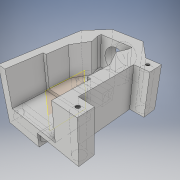
# Autodesk Inventor part: AC_wire_holder
Saved by Autodesk Inventor 2019 (Build 230136000, 136)
## iProperties
Created: 2019-08-30
Part Number: AC_wire_holder
Material: Generic
Document SubType Name: Modeling
Designer: fablab
Density: 1 g/cm^3
Appearance: Default
Author: fablab
Autodesk Inventor part; units mm, degrees
ref_plane "YZ Plane" through (0, 0, 0) normal (1, 0, 0) x (0, 1, 0)
ref_plane "XZ Plane" through (0, 0, 0) normal (0, 1, 0) x (-1, 0, 0)
ref_plane "XY Plane" through (0, 0, 0) normal (0, 0, 1) x (1, 0, 0)
sketch "Sketch1" plane through (0, 0, 0) normal (0, 1, 0) x (-1, 0, 0)
  line L0 (0, 0) -> (-25.32, 0)
  line L1 (-25.32, 0) -> (-25.32, -13)
  line L2 (-25.32, -13) -> (0, -13)
  line L3 (0, -13) -> (0, 0)
  dimension "d0" = 25.32
  dimension "d1" = 13
  constraints: 8 end point, 2 parallel, 1 horizontal, 1 perpendicular
  measures "d0" distance of L2.end L1.end
  measures "d1" distance of L1.end L0.end
extrude "Extrusion1" add sketch "Sketch1" along normal blind 5
sketch "Sketch2" plane through (25.32, 0, 0) normal (1, 0, 0) x (0, 0, -1)
  line L0 (0, 0) -> (13, 0)
  line L1 (13, 0) -> (13, 21.3)
  line L2 (13, 21.3) -> (0, 21.3)
  line L3 (0, 21.3) -> (0, 0)
  dimension "d4" = 13
  dimension "d5" = 21.3
  constraints: 8 end point, 2 parallel, 1 horizontal, 1 perpendicular
  measures "d4" distance of L2.end L1.end
  measures "d5" distance of L1.end L0.end
extrude "Extrusion2" add sketch "Sketch2" along normal blind 7
sketch "Sketch3" plane through (0, 0, 0) normal (0, -1, 0) x (1, 0, 0)
  line L0 (25.32, -13) -> (0, -13) projected
  line L1 (25.32, -8.0084) -> (25.32, -13)
  line L2 (25.32, -13) -> (25.32, -23) construction
  line L3 (25.32, -23) -> (20.12, -23) construction
  line L4 (20.12, -23) -> (25.32, -13)
  line L5 (20.12, -23) -> (5.2, -23)
  line L6 (0, -23) -> (5.2, -23)
  line L7 (5.2, -23) -> (0, -13)
  line L8 (0, -13) -> (5.2, -23)
  point P0 (0, 0)
  dimension "d8" = 10
  dimension "d9" = 5.2
  dimension "d10" = 5.2
  constraints: 16 end point, 2 horizontal, 1 collinear, 1 point on line, 1 vertical
  measures "d8" distance of L0.start L2.end
  measures "d9" distance of L2.end L3.end
  measures "d10" distance of L5.end L6.start
extrude "Extrusion3" add sketch "Sketch3" against normal blind 5
sketch "Sketch4" plane through (0, 0, 0) normal (0, -1, 0) x (1, 0, 0)
  line L0 (20.12, -23) -> (25.32, -13) projected
  line L1 (20.12, -23) -> (27.32, -23)
  line L2 (25.32, -13) -> (32.32, -13) projected
  line L3 (32.32, -13) -> (27.32, -23)
  point P0 (0, 0)
  dimension "d13" = 7.2
  constraints: 4 end point, 1 horizontal
  measures "d13" distance of L0.start L1.end
extrude "Extrusion4" add sketch "Sketch4" against normal blind 21.3
sketch "Sketch5" plane through (0, 0, 0) normal (0, -1, 0) x (1, 0, 0)
  line L0 (20.12, -23) -> (5.2, -23) projected
  line L1 (20.12, -23) -> (20.12, -28.9) construction
  line L2 (20.12, -28.9) -> (22.12, -28.9) construction
  line L3 (20.12, -23) -> (25.32, -13) projected
  line L4 (22.12, -28.9) -> (20.12, -23)
  line L5 (27.32, -23) -> (20.12, -23) projected
  line L6 (27.32, -23) -> (27.32, -28.9)
  line L7 (27.32, -28.9) -> (29.32, -28.9) construction
  line L8 (29.32, -28.9) -> (27.32, -23)
  line L9 (29.32, -28.9) -> (22.12, -28.9)
  line L10 (5.2, -23) -> (5.2, -28.9) construction
  line L11 (5.2, -28.9) -> (3.2, -28.9) construction
  line L12 (3.2, -28.9) -> (5.2, -23)
  line L13 (22.12, -28.9) -> (3.2, -28.9)
  point P0 (0, 0)
  dimension "d16" = 5.9
  dimension "d17" = 2
  dimension "d18" = 2
  dimension "d19" = 2
  constraints: 22 end point, 2 collinear, 2 perpendicular, 2 point on line, 2 vertical, 1 horizontal
  measures "d16" distance of L0.start L1.end
  measures "d17" distance of L1.end L2.end
  measures "d18" distance of L6.end L7.end
  measures "d19" distance of L10.end L11.end
extrude "Extrusion5" add sketch "Sketch5" against normal blind 5 contours L4 L13 L12 L0
sketch "Sketch6" plane through (0, 0, 0) normal (0, -1, 0) x (1, 0, 0)
  line L0 (20.12, -23) -> (27.32, -23) projected
  line L1 (27.32, -23) -> (27.32, -28.9) construction
  line L2 (27.32, -28.9) -> (29.32, -28.9) construction
  line L3 (29.32, -28.9) -> (27.32, -23)
  line L4 (20.12, -23) -> (22.12, -28.9) projected
  line L5 (29.32, -28.9) -> (22.12, -28.9)
  point P0 (0, 0)
  dimension "d22" = 5.9
  dimension "d23" = 2
  constraints: 8 end point, 1 perpendicular, 1 vertical
  measures "d22" distance of L0.end L1.end
  measures "d23" distance of L1.end L2.end
extrude "Extrusion6" add sketch "Sketch6" against normal blind 21.3
sketch "Sketch7" plane through (0, 0, 0) normal (0, -1, 0) x (1, 0, 0)
  line L0 (22.12, -28.9) -> (3.2, -28.9) projected
  line L1 (22.12, -28.9) -> (22.12, -31.4)
  line L2 (3.2, -28.9) -> (5.2, -23) projected
  line L3 (3.2, -28.9) -> (3.2, -31.4)
  line L4 (3.2, -31.4) -> (22.12, -31.4)
  point P0 (0, 0)
  dimension "d26" = 2.5
  dimension "d27" = 2.5
  constraints: 6 end point, 2 vertical
  measures "d26" distance of L0.start L1.end
  measures "d27" distance of L0.end L3.end
extrude "Extrusion7" add sketch "Sketch7" against normal blind 5
sketch "Sketch8" plane through (0, 0, 0) normal (0, -1, 0) x (1, 0, 0)
  line L0 (27.32, -23) -> (29.32, -28.9) projected
  line L1 (22.12, -28.9) -> (22.12, -31.4) projected
  line L2 (29.32, -28.9) -> (22.12, -28.9)
  line L3 (22.12, -28.9) -> (22.12, -31.4)
  line L4 (22.12, -31.4) -> (29.32, -31.4)
  line L5 (29.32, -31.4) -> (29.32, -28.9)
  point P0 (0, 0)
  constraints: 8 end point, 2 parallel, 1 horizontal, 1 perpendicular
extrude "Extrusion8" add sketch "Sketch8" against normal blind 21.3
sketch "Sketch9" plane through (0, 0, 0) normal (0, -1, 0) x (1, 0, 0)
  line L0 (22.12, -31.4) -> (3.2, -31.4) projected
  line L1 (3.2, -31.4) -> (22.12, -31.4)
  line L2 (22.12, -31.4) -> (22.12, -39.7)
  line L3 (22.12, -39.7) -> (3.2, -39.7)
  line L4 (3.2, -39.7) -> (3.2, -31.4)
  point P0 (0, 0)
  dimension "d32" = 18.92
  dimension "d33" = 8.3
  constraints: 8 end point, 2 parallel, 1 horizontal, 1 perpendicular
  measures "d32" distance of L2.end L3.end
  measures "d33" distance of L3.end L0.end
extrude "Extrusion9" add sketch "Sketch9" against normal blind 21.3
sketch "Sketch10" plane through (0, 0, 0) normal (0, -1, 0) x (1, 0, 0)
  line L0 (22.12, -31.4) -> (29.32, -31.4) projected
  line L1 (22.12, -31.4) -> (22.12, -39.7) projected
  line L2 (29.32, -31.4) -> (22.12, -39.7)
  point P0 (0, 0)
  constraints: 2 end point
extrude "Extrusion10" add sketch "Sketch10" against normal blind 21.3
sketch "Sketch11" plane through (3.2, 0, -39.7) normal (0, 0, -1) x (-1, 0, 0)
  line L0 (0, 5) -> (-2, 5) projected
  line L1 (0, 5) -> (-18.878, 5) construction
  line L2 (0, 21.3) -> (-18.92, 21.3) projected
  line L3 (-9.46, 21.3) -> (-9.439, 5) construction
  line L4 (-9.4495, 13.15) -> (0, 13.1622) construction
  line L5 (0, 0) -> (0, 21.3) projected
  circle A0 centre (-9.4495, 13.15) radius 6.625
  point P0 (3.2, 0)
  dimension "d38" = 13.25
  constraints: 6 end point, 3 midpoint, 1 centre point, 1 coincident, 1 collinear, 1 perpendicular, 1 point on line
  measures "d38" diameter of A0
extrude "Extrusion11" cut sketch "Sketch11" against normal blind 21.3
sketch "Sketch12" plane through (25.32, 21.3, 0) normal (0, 1, 0) x (1, 0, 0)
  line L0 (7, 13) -> (2, 23) projected
  line L1 (4, 31.4) -> (4, 28.9) projected
  line L2 (7, 13) -> (4, 31.4)
  line L3 (2, 23) -> (4, 28.9) projected
  line L4 (2, 23) -> (4, 28.9)
  line L5 (4, 28.9) -> (4, 31.4)
  line L6 (7, 13) -> (2, 23)
  point P0 (-25.32, 0)
  constraints: 8 end point, 1 collinear, 1 vertical
extrude "Extrusion12" add sketch "Sketch12" against normal blind 21.3
sketch "Sketch13" plane through (25.32, 21.3, 0) normal (0, 1, 0) x (1, 0, 0)
  line L0 (4, 31.4) -> (7, 13) projected
  line L1 (7, 13) -> (7, 31.4) construction
  line L2 (4, 31.4) -> (7, 27.9417)
  line L3 (4, 31.4) -> (-3.2, 39.7) projected
  line L4 (7, 27.9417) -> (7, 13)
  line L5 (7, 13) -> (4, 31.4)
  point P0 (-25.32, 0)
  constraints: 8 end point, 3 collinear, 1 point on line, 1 vertical
extrude "Extrusion13" add sketch "Sketch13" against normal blind 21.3
ref_plane "Work Plane1" through (12.66, 5, 0) normal (1, 0, 0) x (0, 1, 0)
mirror "Mirror1" about plane through (12.66, 5, 0) normal (1, 0, 0)
sketch "Sketch16" plane through (25.32, 5, 0) normal (0, 0, 1) x (1, 0, 0)
  line L0 (-20.12, 0) -> (-25.32, 0) projected
  line L1 (-25.32, 0) -> (-25.32, -2) construction
  line L2 (-25.32, -2) -> (-27.32, -2)
  line L3 (-27.32, -2) -> (-27.32, 16.3)
  line L4 (-25.32, 16.3) -> (-32.32, 16.3) projected
  line L5 (0, 0) -> (2, 0) construction
  line L6 (2, 0) -> (2, -2)
  line L7 (2, -2) -> (-25.32, -2)
  line L8 (2, 0) -> (2, 16.3)
  line L9 (-27.32, 16.3) -> (-32.32, 16.3)
  line L10 (-32.32, 16.3) -> (-32.32, -5) projected
  line L11 (-32.32, 16.3) -> (-32.32, -5)
  line L12 (-32.32, -5) -> (7, -5)
  line L13 (7, 16.3) -> (7, -5) projected
  line L14 (7, -5) -> (7, 16.3)
  line L15 (7, 16.3) -> (2, 16.3)
  line L16 (0, 16.3) -> (7, 16.3) projected
  point P0 (-25.32, -5)
  dimension "d45" = 2
  dimension "d46" = 2
  dimension "d47" = 2
  dimension "d48" = 2
  constraints: 24 end point, 4 perpendicular, 3 collinear, 2 horizontal, 2 point on line, 1 vertical
  measures "d45" distance of L0.end L1.end
  measures "d46" distance of L1.end L2.end
  measures "d47" distance of L5.start L5.end
  measures "d48" distance of L5.end L6.end
extrude "Extrusion14" add sketch "Sketch16" along normal blind 19.2
sketch "Sketch22" plane through (-7, 0, -27.9417) normal (-1, 0, 0) x (0, 0, 1)
  line L0 (-11.7583, 0) -> (0, 0) projected
  line L1 (0, 0) -> (8, 0)
  line L2 (8, 0) -> (8, -8)
  line L3 (8, -8) -> (0, -8)
  line L4 (0, -8) -> (0, 0)
  line L5 (47.1417, 0) -> (0, 0) projected
  line L6 (47.1417, 0) -> (39.1417, 0)
  line L7 (39.1417, 0) -> (39.1417, -8)
  line L8 (39.1417, -8) -> (47.1417, -8)
  line L9 (47.1417, -8) -> (47.1417, 0)
  line L10 (0, -4) -> (47.1417, -4) construction
  line L11 (4, -8) -> (4, -4) construction
  line L12 (43.1417, -8) -> (43.1417, -4) construction
  circle A0 centre (4, -4) radius 1
  circle A1 centre (43.1417, -4) radius 1
  point P0 (27.9417, 0)
  dimension "d81" = 8
  dimension "d82" = 8
  dimension "d83" = 8
  dimension "d84" = 8
  dimension "d85" = 2
  dimension "d86" = 2
  constraints: 22 end point, 4 midpoint, 4 parallel, 4 perpendicular, 2 centre point, 2 coincident, 2 horizontal, 2 point on line
  measures "d81" distance of L2.end L3.end
  measures "d82" distance of L1.end L2.end
  measures "d83" distance of L8.end L7.end
  measures "d84" distance of L7.end L6.end
  measures "d85" diameter of A0
  measures "d86" diameter of A1
extrude "Extrusion20" add sketch "Sketch22" against normal blind 2.5
chamfer "Chamfer2" distance 2 angle 45 2 edges at (-4.5, -4, -24.9417) (-4.5, -4, 14.2)
sketch "Sketch24" plane through (25.32, 21.3, 0) normal (0, 1, 0) x (1, 0, 0)
  line L0 (-27.32, -19.2) -> (-32.32, -19.2) projected
  line L1 (-27.32, -19.2) -> (-32.32, -19.2)
  line L2 (-32.32, 27.9417) -> (-32.32, -19.2) projected
  line L3 (-32.32, -19.2) -> (-32.32, 27.9417)
  line L4 (-32.32, 27.9417) -> (-22.12, 39.7) projected
  line L5 (-32.32, 27.9417) -> (-22.12, 39.7)
  line L6 (-3.2, 39.7) -> (-22.12, 39.7) projected
  line L7 (-22.12, 39.7) -> (-3.2, 39.7)
  line L8 (-3.2, 39.7) -> (7, 27.9417)
  line L9 (7, -19.2) -> (7, 27.9417) projected
  line L10 (7, 27.9417) -> (7, -19.2)
  line L11 (7, -19.2) -> (2, -19.2) projected
  line L12 (7, -19.2) -> (2, -19.2)
  line L13 (0, 0) -> (2, 0) projected
  line L14 (2, -19.2) -> (2, 0)
  line L15 (2, 0) -> (0, 0)
  line L16 (0, 13) -> (0, 0) projected
  line L17 (0, 0) -> (0, 13)
  line L18 (-5.2, 23) -> (0, 13) projected
  line L19 (0, 13) -> (-5.2, 23)
  line L20 (-3.2, 28.9) -> (-5.2, 23) projected
  line L21 (-5.2, 23) -> (-3.2, 28.9)
  line L22 (-3.2, 28.9) -> (-3.2, 31.4)
  line L23 (-22.12, 31.4) -> (-3.2, 31.4) projected
  line L24 (-3.2, 31.4) -> (-22.12, 31.4)
  line L25 (-22.12, 31.4) -> (-22.12, 28.9) projected
  line L26 (-22.12, 31.4) -> (-22.12, 28.9)
  line L27 (-22.12, 28.9) -> (-20.12, 23) projected
  line L28 (-22.12, 28.9) -> (-20.12, 23)
  line L29 (-20.12, 23) -> (-25.32, 13) projected
  line L30 (-20.12, 23) -> (-25.32, 13)
  line L31 (-25.32, 13) -> (-25.32, 0) projected
  line L32 (-25.32, 13) -> (-25.32, 0)
  line L33 (-25.32, 0) -> (-27.32, 0) projected
  line L34 (-25.32, 0) -> (-27.32, 0)
  line L35 (-27.32, 0) -> (-27.32, -19.2) projected
  line L36 (-27.32, 0) -> (-27.32, -19.2)
  line L37 (-25.32, 13) -> (-25.32, 0) projected
  line L38 (0, 0) -> (-25.32, 0)
  constraints: 42 end point, 12 collinear, 4 perpendicular, 2 horizontal, 2 parallel
extrude "Extrusion22" add sketch "Sketch24" along normal blind 2 contours L0 L2 L4 L6 L8 L9 L11 L14 L13 L16 L18 L20 L22 L23 L25 L27 L29 L31 L33 L35
sketch "Sketch25" plane through (25.32, 23.3, 0) normal (0, 1, 0) x (1, 0, 0)
  line L0 (2, -19.2) -> (7, -19.2) projected
  line L1 (7, -19.2) -> (15, -19.2)
  line L2 (15, -19.2) -> (15, -11.2)
  line L3 (15, -11.2) -> (7, -11.2)
  line L4 (7, -11.2) -> (7, -19.2)
  line L5 (7, -19.2) -> (7, 27.9417) projected
  line L6 (7, 27.9417) -> (15, 27.9417)
  line L7 (15, 27.9417) -> (15, 19.9417)
  line L8 (15, 19.9417) -> (7, 19.9417)
  line L9 (7, 19.9417) -> (7, 27.9417)
  line L10 (11, -19.2) -> (11, 27.9417) construction
  line L11 (15, -15.2) -> (11, -15.2) construction
  line L12 (15, 23.9417) -> (11, 23.9417) construction
  circle A0 centre (11, -15.2) radius 1
  circle A1 centre (11, 23.9417) radius 1
  point P0 (-25.32, 0)
  dimension "d96" = 8
  dimension "d97" = 8
  dimension "d98" = 8
  dimension "d99" = 8
  dimension "d100" = 2
  dimension "d101" = 2
  constraints: 22 end point, 4 midpoint, 4 parallel, 4 perpendicular, 2 centre point, 2 coincident, 2 horizontal, 2 point on line
  measures "d96" distance of L3.end L2.end
  measures "d97" distance of L2.end L1.end
  measures "d98" distance of L7.end L8.end
  measures "d99" distance of L6.end L7.end
  measures "d100" diameter of A0
  measures "d101" diameter of A1
extrude "Extrusion23" add sketch "Sketch25" against normal blind 2
chamfer "Chamfer3" distance 2 angle 45 2 edges at (35.32, 21.3, 15.2) (35.32, 21.3, -23.9417)
sketch "Sketch26" plane through (25.32, 21.3, 0) normal (0, -1, 0) x (1, 0, 0)
  circle A0 centre (11, 15.2) radius 1 projected
  circle A1 centre (11, 15.2) radius 3 projected
  line L0 (15, 19.2) -> (7, 19.2) projected
  line L1 (7, 11.2) -> (7, 19.2) projected
  line L2 (7, 11.2) -> (15, 11.2) projected
  line L3 (15, 11.2) -> (15, 19.2) projected
  circle A2 centre (11, 15.2) radius 3 projected
  circle A3 centre (11, 15.2) radius 3
  line L4 (15, 19.2) -> (7, 19.2) projected
  line L5 (15, 19.2) -> (7, 19.2)
  line L6 (7, 19.2) -> (7, 11.2)
  line L7 (7, 11.2) -> (15, 11.2)
  line L8 (15, 11.2) -> (15, 19.2)
  point P0 (-25.32, 0)
  constraints: 8 end point, 2 parallel, 1 centre point, 1 coincident, 1 concentric, 1 horizontal, 1 perpendicular
extrude "Extrusion24" add sketch "Sketch26" along normal blind 21.3 contours L3 L2 L1 L0
sketch "Sketch28" plane through (25.32, 21.3, 0) normal (0, -1, 0) x (1, 0, 0)
  circle A0 centre (11, -23.9417) radius 1 projected
  circle A1 centre (11, -23.9417) radius 3 projected
  line L0 (7, -27.9417) -> (7, -19.9417) projected
  line L1 (7, -27.9417) -> (15, -27.9417) projected
  line L2 (15, -27.9417) -> (15, -19.9417) projected
  line L3 (15, -19.9417) -> (7, -19.9417) projected
  circle A2 centre (11, -23.9417) radius 3 projected
  circle A3 centre (11, -23.9417) radius 3
  line L4 (7, -27.9417) -> (-3.2, -39.7) projected
  line L5 (15, -19.9417) -> (15, -27.9417) projected
  line L6 (7, -27.9417) -> (15, -27.9417)
  line L7 (15, -27.9417) -> (15, -19.9417)
  line L8 (15, -19.9417) -> (7, -19.9417)
  line L9 (7, -19.9417) -> (7, -27.9417)
  point P0 (-25.32, 0)
  constraints: 8 end point, 2 parallel, 1 centre point, 1 coincident, 1 concentric, 1 horizontal, 1 perpendicular
extrude "Extrusion25" add sketch "Sketch28" along normal blind 21.3 contours L0 L3 L2 L1
sketch "Sketch29" plane through (-4.5, 0, -27.9417) normal (1, 0, 0) x (0, 0, -1)
  circle A0 centre (-43.1417, -4) radius 1 projected
  circle A1 centre (-43.1417, -4) radius 3 projected
  line L0 (-47.1417, 0) -> (-39.1417, 0) projected
  line L1 (-47.1417, 0) -> (-47.1417, -8) projected
  line L2 (-47.1417, -8) -> (-39.1417, -8) projected
  line L3 (-39.1417, -8) -> (-39.1417, 0) projected
  circle A2 centre (-43.1417, -4) radius 3 projected
  circle A3 centre (-4, -4) radius 1 projected
  circle A4 centre (-4, -4) radius 3 projected
  line L4 (0, -8) -> (0, 0) projected
  line L5 (-8, 0) -> (0, 0) projected
  line L6 (-8, 0) -> (-8, -8) projected
  line L7 (-8, -8) -> (0, -8) projected
  circle A5 centre (-4, -4) radius 3 projected
  line L8 (-39.1417, -8) -> (-47.1417, -8)
  line L9 (-47.1417, -8) -> (-47.1417, 0)
  line L10 (-47.1417, 0) -> (-39.1417, 0)
  line L11 (-39.1417, 0) -> (-39.1417, -8)
  line L12 (-8, -8) -> (0, -8) projected
  line L13 (0, -8) -> (-8, -8)
  line L14 (-8, -8) -> (-8, 0)
  line L15 (-8, 0) -> (0, 0)
  line L16 (0, 0) -> (0, -8)
  circle A6 centre (-43.1417, -4) radius 3
  circle A7 centre (-4, -4) radius 1 projected
  circle A8 centre (-4, -4) radius 3
  point P0 (-27.9417, 0)
  constraints: 16 end point, 4 parallel, 2 centre point, 2 coincident, 2 concentric, 2 horizontal, 2 perpendicular
extrude "Extrusion26" add sketch "Sketch29" along normal blind 20 contours L0 L3 L2 L1 | L7 L6 L5 L4
body "Solid1"
